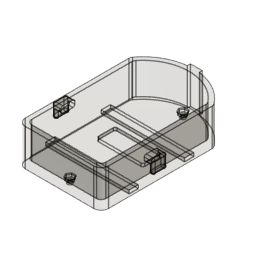
RyobiBatteryHolder v7 (Autodesk Fusion 360 design; units mm, degrees)
Autodesk Fusion 360 part; units mm, degrees
sketch "Sketch1" plane through (0, 0, 0) normal (0, 0, 1) x (1, 0, 0)
  line L0 (0, 0) -> (80, 0)
  line L1 (80, 0) -> (80, 135) construction
  line L2 (0, 135) -> (0, 0) construction
  line L3 (0, 135) -> (80, 135) construction
  line L4 (80, 135) -> (80, 115) construction
  line L5 (80, 115) -> (0, 115) construction
  arc A0 (80, 115) -> (0, 115) centre (40, 85) ccw
  line L6 (0, 0) -> (0, 115)
  line L7 (80, 115) -> (80, 0)
  line L8 (-5, -5) -> (85, -5)
  line L9 (85, 116.6228) -> (85, -5)
  arc A1 (85, 116.6228) -> (-5, 116.6228) centre (40, 85) ccw
  line L10 (-5, -5) -> (-5, 116.6228)
  line L11 (33.5, 143) -> (46.5, 143)
  line L12 (46.5, 143) -> (46.5, 135)
  line L13 (46.5, 135) -> (33.5, 135)
  line L14 (33.5, 135) -> (33.5, 143)
  line L15 (85, -5) -> (58.74, -5) construction
  line L16 (85, 41.4) -> (85, -5) construction
  circle A2 centre (167.6575, 118.9529) radius 2.1
  line L17 (65, 60.1571) -> (15, 60.1571)
  line L18 (15, 60.1571) -> (15, 80.1571)
  line L19 (15, 80.1571) -> (65, 80.1571)
  line L20 (65, 80.1571) -> (65, 60.1571)
  line L21 (15, 80.1571) -> (65, 60.1571) construction
  line L22 (15, 60.1571) -> (65, 80.1571) construction
  line L23 (40, 70.1571) -> (40, 159.8429) construction
  line L24 (-17.6351, 6.3905) -> (104.3649, 6.3905) construction
  line L25 (104.3649, 6.3905) -> (104.3649, 128.3905) construction
  line L26 (104.3649, 128.3905) -> (-17.6351, 128.3905) construction
  line L27 (-17.6351, 128.3905) -> (-17.6351, 6.3905) construction
  line L28 (40, 85) -> (40, -59.4734) construction
  circle A3 centre (40, 6.3905) radius 2
  circle A4 centre (40, 128.3905) radius 2
  circle A5 centre (40, 6.3905) radius 3.55 construction
  circle A6 centre (40, 128.3905) radius 3.55 construction
  line L29 (35.9013, 6.4524) -> (37.8971, 2.8718)
  line L30 (37.8971, 2.8718) -> (41.9958, 2.81)
  line L31 (41.9958, 2.81) -> (44.0987, 6.3287)
  line L32 (44.0987, 6.3287) -> (42.1029, 9.9092)
  line L33 (42.1029, 9.9092) -> (38.0042, 9.971)
  line L34 (38.0042, 9.971) -> (35.9013, 6.4524)
  line L35 (42.1765, 131.8642) -> (38.0799, 132.0122)
  line L36 (38.0799, 132.0122) -> (35.9035, 128.5385)
  line L37 (35.9035, 128.5385) -> (37.8235, 124.9168)
  line L38 (37.8235, 124.9168) -> (41.9201, 124.7688)
  line L39 (41.9201, 124.7688) -> (44.0965, 128.2425)
  line L40 (44.0965, 128.2425) -> (42.1765, 131.8642)
  point P0 (74.4902, 112.6066)
  point P1 (40, 6.3905)
  point P2 (40, 128.3905)
  dimension "d1" = 80
  dimension "d2" = 135
  dimension "d3" = 20
  dimension "d4" = -5
  dimension "d9" = 13
  dimension "d10" = 8
  dimension "d44" = 26.26
  dimension "d45" = 46.4
  dimension "d48" = 4.2
  dimension "d49" = 50
  dimension "d50" = 20
  dimension "d75" = 122
  dimension "d76" = 122
  dimension "d77" = 4
  dimension "d78" = 4
  dimension "d79" = 7.1
  dimension "d80" = 7.1
  constraint horizontal L0
  constraint vertical L1
  constraint vertical L2
  constraint coincident L0.start L2.end
  constraint horizontal L3
  constraint vertical L4
  constraint horizontal L5
  constraint tangent L3 A0
  constraint perpendicular L5 L6
  constraint perpendicular L0 L7
  constraint horizontal L11
  constraint vertical L12
  constraint horizontal L13
  constraint vertical L14
  constraint midpoint A0 L13
  constraint horizontal L15
  constraint vertical L16
  constraint coincident L8.end L9.end
  constraint horizontal L17
  constraint vertical L18
  constraint horizontal L19
  constraint vertical L20
  constraint midpoint L21 L23.start
  constraint perpendicular L19 L23
  constraint midpoint L5 L23
  constraint horizontal L24
  constraint vertical L25
  constraint horizontal L26
  constraint vertical L27
  constraint coincident A0.centre A1.centre
  constraint perpendicular L19 L28
  constraint coincident L28 P1
  constraint coincident L24 P1
  constraint coincident L23 P2
  constraint coincident L26 P2
  constraint concentric A3 A5
  constraint concentric A4 A6
  constraint coincident P1 A3.centre
  constraint coincident P2 A4.centre
  measures "d1" distance of L0.start L0.end
  measures "d2" distance of L0.start L2.start
  measures "d3" distance of L2.start L5.end
  measures "d9" distance of L11.start L11.end
  measures "d10" distance of L11.start L13.end
  measures "d44" distance of L8.end L15.end
  measures "d45" distance of L8.end L16.start
  measures "d48" diameter of A2
  measures "d49" distance of L17.start L17.end
  measures "d50" distance of L17.start L19.end
  measures "d75" distance of L24.start L24.end
  measures "d76" distance of L24.start L26.end
  measures "d77" diameter of A3
  measures "d78" diameter of A4
  measures "d79" diameter of A5
  measures "d80" diameter of A6
extrude "Floor" add sketch "Sketch1" along normal blind 6 contours L0 A0 L6 L7 | L8 L9 A1 L10 L12 L13 L14 | A1 L12 L13 L14 | L17 L18 L19 L20 | A3 | A4 | L29 L30 L31 L32 L33 L34 | L35 L36 L37 L38 L39 L40 makes body 1
extrude "Sides" add sketch "Sketch1" along normal blind 40 contours L8 L9 A1 L10 L12 L13 L14 | A1 L12 L13 L14 bodies 1
extrude "Extrude3" add sketch "Sketch1" along normal blind 40 contours A1 L12 L13 L14 | A1 L11 L12 L14 bodies 1
sketch "Sketch3" plane through (-5, 0, 0) normal (-1, 0, 0) x (0, -1, 0)
  line L0 (-116.6228, 0) -> (5, 0)
  line L1 (5, 0) -> (5, 40)
  line L2 (5, 40) -> (-116.6228, 40)
  line L3 (-116.6228, 40) -> (-116.6228, 0)
  line L4 (-95.0874, 6.3184) -> (-85.0874, 6.3184)
  line L5 (-85.0874, 6.3184) -> (-85.0874, 2.8184)
  line L6 (-85.0874, 2.8184) -> (-95.0874, 2.8184)
  line L7 (-95.0874, 2.8184) -> (-95.0874, 6.3184)
  line L8 (-35.0874, 2.8184) -> (-35.0874, 6.3184)
  line L9 (-25.0874, 6.3184) -> (-25.0874, 2.8184)
  line L10 (-35.0874, 6.3184) -> (-25.0874, 6.3184)
  line L11 (-25.0874, 2.8184) -> (-35.0874, 2.8184)
  line L12 (-93.2742, 68.1482) -> (-78.2742, 68.1482)
  line L13 (-78.2742, 68.1482) -> (-78.2742, 53.1482)
  line L14 (-78.2742, 53.1482) -> (-93.2742, 53.1482)
  line L15 (-93.2742, 53.1482) -> (-93.2742, 68.1482)
  line L16 (-93.2742, 68.1482) -> (-78.2742, 68.1482)
  line L17 (-78.2742, 68.1482) -> (-78.2742, 61.1482)
  line L18 (-78.2742, 61.1482) -> (-93.2742, 61.1482)
  line L19 (-93.2742, 61.1482) -> (-93.2742, 68.1482)
  dimension "d25" = 10
  dimension "d26" = 3.5
  dimension "d27" = 10
  dimension "d28" = 3.5
  dimension "d64" = 15
  dimension "d65" = 15
  dimension "d66" = 7
  constraint horizontal L4
  constraint vertical L5
  constraint horizontal L6
  constraint vertical L7
  constraint horizontal L10
  constraint vertical L9
  constraint horizontal L11
  constraint vertical L8
  constraint horizontal L12
  constraint vertical L13
  constraint horizontal L14
  constraint vertical L15
  constraint horizontal L16
  constraint vertical L17
  constraint horizontal L18
  constraint vertical L19
  measures "d25" distance of L4.start L4.end
  measures "d26" distance of L4.start L6.end
  measures "d27" distance of L9.start L8.end
  measures "d28" distance of L8.start L8.end
  measures "d64" distance of L12.start L12.end
  measures "d65" distance of L12.start L14.end
  measures "d66" distance of L12.start L18.end
extrude "CutSlotsOnBottom" cut sketch "Sketch3" against normal blind 100 contours L4 L5 L6 L7 | L8 L9 L10 L11 bodies 1
extrude "Extrude9" cut sketch "Sketch1" along normal blind 3.2 contours L17 L18 L19 L20 bodies 1
fillet "Fillet1" radius 2 4 edges at (15, 60.1571, 1.6) (65, 60.1571, 1.6) (65, 80.1571, 1.6) (15, 80.1571, 1.6) on bodies 1
fillet "Fillet2" radius 5 2 edges at (0, 0, 23) (80, 0, 23) on bodies 1
fillet "Fillet3" radius 8 2 edges at (85, -5, 20) (-5, -5, 20) on bodies 1
fillet "Fillet4" radius 5 2 edges at (0, 115, 23) (80, 115, 23) on bodies 1
fillet "Fillet5" radius 5 2 edges at (85, 116.6228, 20) (-5, 116.6228, 20) on bodies 1
extrude "Extrude10" add sketch "Sketch3" along normal blind 10 separate body contours L12 L13 L15 L16 L17 L18 L19 makes body 2
extrude "Extrude11" add sketch "Sketch3" along normal blind 5 contours L13 L14 L15 L18 bodies 2
fillet "Fillet6" radius 2 12 edges at (-5, 93.2742, 60.6482) (-5, 85.7742, 68.1482) (-5, 78.2742, 60.6482) (-5, 85.7742, 53.1482) (-10, 93.2742, 68.1482) (-10, 78.2742, 68.1482) (-12.5, 93.2742, 61.1482) (-10, 93.2742, 57.1482) (-7.5, 93.2742, 53.1482) (-7.5, 78.2742, 53.1482) (-12.5, 78.2742, 61.1482) (-10, 78.2742, 57.1482) on bodies 2
move_body "Move1" bodies 2 to x (1, 0, 0) y (0, 1, 0) z (0, 0, 1) at (100.1268, -36.7132, 0)
copy_body "CopyPasteBodies1" bodies 2 makes body 3
move_body "Move2" bodies 3 to x (-1, 0, 0) y (0, -1, 0) z (0, 0, 1) at (79.9787, 98.122, 0)
move_body "Move3" bodies 3 2 to x (1, 0, 0) y (0, 1, 0) z (0, 0, 1) at (0, 0, -37.2216)
fillet "Fillet7" radius 2 6 edges at (90.7126, 55.9752, 16.5124) (90.1268, 49.061, 15.9266) (90.7126, 42.1468, 16.5124) (-10.7339, 42.1468, 16.5124) (-10.1481, 49.061, 15.9266) (-10.7339, 55.9752, 16.5124) on bodies 2 3
move_body "Move4" bodies 3 to x (1, 0, 0) y (0, 1, 0) z (0, 0, 1) at (0.3239, 0, 0)
move_body "Move5" bodies 2 to x (1, 0, 0) y (0, 1, 0) z (0, 0, 1) at (-0.2944, 0, 0)
combine "Combine1" operation add target body 1 tool bodies 3 2
extrude "Extrude12" cut sketch "Sketch1" against normal blind 3.2 from surface at 6 contours L29 L30 L31 L32 L33 L34 | L35 L36 L37 L38 L39 L40 bodies 1
extrude "Extrude13" cut 2 faces at (39.8517, 7.0405, 6) (40.4961, 128.9433, 6) along direction (0, 0, -1) blind 8 on bodies 1 bodies 1
chamfer "Chamfer2" distance 0.75 angle 45 14 edges at (36.9527, 8.2117, 6) (40.0536, 9.9401, 6) (43.1008, 8.1189, 6) (43.0473, 4.5693, 6) (39.9464, 2.8409, 6) (36.8992, 4.6621, 6) (36.8635, 126.7277, 6) (36.9917, 130.2754, 6) (40.1282, 131.9382, 6) (43.1365, 130.0533, 6) (43.0083, 126.5057, 6) (39.8718, 124.8428, 6) (38.1353, 5.6673, 0) (38.1353, 127.6673, 0) on bodies 1
